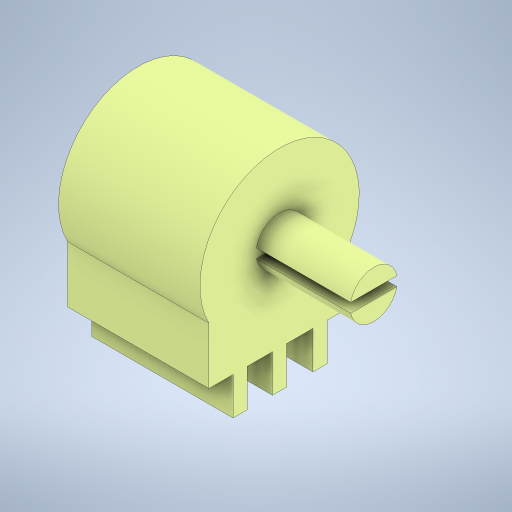
# Autodesk Inventor part: 가변저항
Saved by Autodesk Inventor 2024 (Build 280153000, 153)
## iProperties
Created: 2024-04-21
Part Number: 가변저항
Material: 일반
Document SubType Name: Modeling
Designer: kkamin5
Density: 1 g/cm^3
Appearance: 기본값
Mass: 4.39974 g
Surface Area: 20.8656 cm^2
Volume: 4.39974 cm^3
Author: kkamin5
Autodesk Inventor part; units mm, degrees
ref_plane "YZ Plane" through (0, 0, 0) normal (1, 0, 0) x (0, 1, 0)
ref_plane "XZ Plane" through (0, 0, 0) normal (0, 1, 0) x (-1, 0, 0)
ref_plane "XY Plane" through (0, 0, 0) normal (0, 0, 1) x (1, 0, 0)
sketch "스케치1" plane through (0, 0, 0) normal (1, 0, 0) x (0, 1, 0)
  circle A0 centre (0, 0) radius 8.45
  dimension "d0" = 16.9
  constraints: 1 centre point, 1 coincident
  measures "d0" diameter of A0
extrude "돌출1" add sketch "스케치1" along normal blind 15
sketch "스케치2" plane through (15, 0, 0) normal (1, 0, 0) x (0, 0, -1)
  circle A0 centre (0, 0) radius 2.5
  line L0 (-2.4495, 0.5) -> (2.4495, 0.5)
  line L1 (-2.4495, -0.5) -> (2.4495, -0.5)
  point P0 (0, 0.5)
  dimension "d3" = 5
  dimension "d4" = 1
  dimension "d5" = 0.5
  constraints: 4 end point, 4 point on circle, 1 centre point, 1 coincident, 1 horizontal, 1 midpoint, 1 parallel
  measures "d3" diameter of A0
  measures "d4" distance from line of L1 point (0, 0.5)
  measures "d5" distance from line of point (0, 0) L0
extrude "돌출2" add sketch "스케치2" along normal blind 10 contours L0 A0 | A0 L1
sketch "스케치3" plane through (0, 0, 0) normal (-1, 0, 0) x (0, 0, 1)
  line L0 (-7.5, -3.8926) -> (7.5, -3.8926)
  line L1 (7.5, -3.8926) -> (7.5, -9.8926)
  line L2 (7.5, -9.8926) -> (-7.5, -9.8926)
  line L3 (-7.5, -9.8926) -> (-7.5, -3.8926)
  circle A0 centre (0, 0) radius 8.45 projected
  line L4 (-5.0426, -9.8926) -> (-3.5426, -9.8926)
  line L5 (-3.5426, -9.8926) -> (-3.5426, -13.8926)
  line L6 (-3.5426, -13.8926) -> (-5.0426, -13.8926)
  line L7 (-5.0426, -13.8926) -> (-5.0426, -9.8926)
  line L8 (-0.7464, -9.8926) -> (0.7536, -9.8926)
  line L9 (0.7536, -9.8926) -> (0.7536, -13.8926)
  line L10 (0.7536, -13.8926) -> (-0.7464, -13.8926)
  line L11 (-0.7464, -13.8926) -> (-0.7464, -9.8926)
  line L12 (3.4319, -9.8926) -> (4.9319, -9.8926)
  line L13 (4.9319, -9.8926) -> (4.9319, -13.8926)
  line L14 (4.9319, -13.8926) -> (3.4319, -13.8926)
  line L15 (3.4319, -13.8926) -> (3.4319, -9.8926)
  point P0 (0.7536, -9.8926)
  dimension "d8" = 6
  dimension "d9" = 15
  dimension "d10" = 4
  dimension "d11" = 4
  dimension "d12" = 1.5
  dimension "d13" = 1.5
  dimension "d14" = 1.5
  constraints: 32 end point, 8 parallel, 4 horizontal, 4 perpendicular, 4 point on line, 2 point on circle
  measures "d8" distance of L2.end L0.start
  measures "d9" distance of L1.end L2.end
  measures "d10" distance of L6.end L4.start
  measures "d11" distance of L10.end L8.start
  measures "d12" distance of L9.end L10.end
  measures "d13" distance of L13.end L14.end
  measures "d14" distance of L5.end L6.end
extrude "돌출3" add sketch "스케치3" against normal blind 15 contours A0 L1 L2 L3 | L2 L5 L6 L7 | L13 L14 L15 L2 | L2 L9 L10 L11
equation "\"d11\" = d10"
equation "\"d13\" = d12"
equation "\"d14\" = d12"
